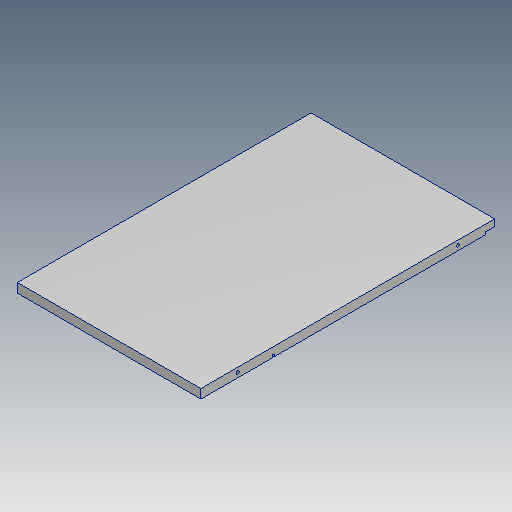
# Autodesk Inventor part: topBottom
Saved by Autodesk Inventor 2017 (Build 210142000, 142)
## iProperties
Created: 2015-10-13
Part Number: topBottom
Material: Aluminum 6061
Document SubType Name: Modeling
Designer: Sawaiz
Density: 2.7 g/cm^3
Appearance: Aluminum - Flat
Mass: 409.812 g
Surface Area: 530.642 cm^2
Volume: 151.782 cm^3
Author: Sawaiz
Autodesk Inventor part; units mm, degrees
ref_plane "YZ Plane" through (0, 0, 0) normal (1, 0, 0) x (0, 1, 0)
ref_plane "XZ Plane" through (0, 0, 0) normal (0, 1, 0) x (-1, 0, 0)
ref_plane "XY Plane" through (0, 0, 0) normal (0, 0, 1) x (1, 0, 0)
sketch "Sketch1" plane through (0, 0, 0) normal (0, 0, 1) x (1, 0, 0)
  line L0 (-101.6, -63.5) -> (101.6, -63.5)
  line L1 (101.6, -63.5) -> (101.6, 63.5)
  line L2 (101.6, 63.5) -> (-101.6, 63.5)
  line L3 (-101.6, 63.5) -> (-101.6, -63.5)
  line L4 (-101.6, -63.5) -> (101.6, 63.5) construction
  line L5 (101.6, -63.5) -> (-101.6, 63.5) construction
  point P0 (0, 0)
  dimension "d0" = 203.2
  dimension "d1" = 127
  constraints: 12 end point, 2 midpoint, 2 parallel, 1 horizontal, 1 perpendicular
  measures "d0" distance of L2.end L1.end
  measures "d1" distance of L1.end L0.end
extrude "Extrusion1" add sketch "Sketch1" along normal blind 6.35
sketch "Sketch16" plane through (0, 0, 0) normal (0, 0, -1) x (-1, 0, 0)
  line L0 (-101.6, 63.5) -> (101.6, 63.5) projected
  line L1 (101.6, -63.5) -> (-101.6, -63.5) projected
  line L2 (-52.3875, 63.5) -> (-50.8, 63.5)
  line L3 (-50.8, 63.5) -> (-50.8, -63.5)
  line L4 (-50.8, -63.5) -> (-52.3875, -63.5)
  line L5 (-52.3875, -63.5) -> (-52.3875, 63.5)
  line L6 (-101.6, -63.5) -> (-101.6, 63.5) projected
  point P0 (0, 0)
  dimension "d114" = 1.5875
  dimension "d115" = 49.2125
  constraints: 8 end point, 2 parallel, 2 point on line, 1 horizontal, 1 perpendicular
  measures "d114" distance between parallel lines of L3 L5
  measures "d115" distance between parallel lines of L6 L5
extrude "Extrusion9" cut sketch "Sketch16" against normal blind 1.6891 contours L0 L3 L1 L5
sketch "Sketch17" plane through (-101.6, 63.5, 6.35) normal (0, 1, 0) x (1, 0, 0)
  line L0 (153.9875, 6.35) -> (153.9875, 4.6609) projected
  line L1 (153.9875, 4.6609) -> (152.4, 4.6609) projected
  line L2 (152.4, 4.6609) -> (152.4, 6.35) projected
  line L3 (152.4, 6.35) -> (0, 6.35) projected
  line L4 (0, 6.35) -> (0, 0) projected
  line L5 (203.2, 0) -> (0, 0) projected
  line L6 (203.2, 6.35) -> (203.2, 0) projected
  line L7 (203.2, 6.35) -> (153.9875, 6.35) projected
  point P0 (101.6, 6.35)
  point P1 (177.8, 3.175)
  point P2 (25.4, 3.175)
  dimension "d118" = 25.4
  dimension "d119" = 25.4
  dimension "d120" = 3.175
  dimension "d121" = 3.175
  measures "d118" distance from line of L4 point (25.4, 3.175)
  measures "d119" distance from line of L6 point (177.8, 3.175)
  measures "d120" distance from line of L5 point (177.8, 3.175)
  measures "d121" distance from line of L5 point (25.4, 3.175)
hole "Hole7" at (76.2, 63.5, 3.175) at (-76.2, 63.5, 3.175) direction (0, -1, 0) diameter 2.159 depth 8.8646 tip angle 118
mirror "Mirror5" about plane through (0, 0, 0) normal (0, 1, 0) of "Hole7"
sketch "Sketch18" plane through (0, 0, 0) normal (0, 0, -1) x (-1, 0, 0)
  line L0 (-50.8, 63.5) -> (-50.8, -63.5) projected
  line L1 (101.6, -63.5) -> (-50.8, -63.5) projected
  line L2 (101.6, 63.5) -> (101.6, -63.5) projected
  line L3 (-50.8, 63.5) -> (101.6, 63.5) projected
  line L4 (-101.6, 63.5) -> (101.6, 63.5) projected
  line L5 (95.1992, 63.5) -> (101.6508, 63.5)
  line L6 (101.6508, 63.5) -> (101.6508, -63.5)
  line L7 (101.6508, -63.5) -> (95.1992, -63.5)
  line L8 (95.1992, -63.5) -> (95.1992, 63.5)
  point P0 (0, 0)
  dimension "d129" = 6.4516
  dimension "d130" = 152.4508
  constraints: 8 end point, 2 parallel, 2 point on line, 1 horizontal, 1 perpendicular
  measures "d129" distance between parallel lines of L8 L6
  measures "d130" distance between parallel lines of L0 L6
extrude "Extrusion10" cut sketch "Sketch18" against normal blind 1.6891 contours L3 L2 L1 L8 | L5 L6 L7 L2
equation "\"width\" = 127"
equation "\"depth\" = 203.2"
equation "\"aerogelHolderDepth\" = 49.2125"
equation "\"caseThickness\" = 6.35"
equation "\"alignmentGrooveDepth\" = 1.5875"
equation "\"height\" = 127"
equation "\"mirrorAngle\" = 2.5deg"
equation "\"mirrorThickness\" = 3.175"
equation "\"fresnelThickness\" = 0.254"
equation "\"focalLength\" = 152.4"
equation "\"ior\" = 1.49"
equation "\"centerThickness\" = 1.27"
equation "\"fresnelAngle\" = 90deg"
equation "\"fresnelEffectiveDiameter\" = 152.4"
equation "\"alignmentGrooveClearance\" = 0.1016"
equation "\"frontPanelThickness\" = 1.5875"
body "Solid1"
